Autodesk Fusion 360 part; units mm, degrees
note: some values were not read from the file. Chosen so that the rebuilt part matches the saved one: which face or edge a step refers to. Set by a fixed rule: which sketch regions a step uses.
(part 2 of 2)
sketch "Cap IV" plane through (0, 0, 30.6) normal (0, 0, 1) x (-1, 0, 0)
  circle A0 centre (-1.55, -2.515) radius 7.04 construction
  circle A1 centre (-1.55, -2.515) radius 7.405
  circle A2 centre (-1.55, -2.515) radius 7.24
  line L0 (5.6884, -2.365) -> (5.8535, -2.365) construction
  line L1 (5.69, -2.515) -> (5.855, -2.515) construction
  line L2 (5.6884, -2.665) -> (5.8535, -2.665) construction
  line L3 (-8.9535, -2.665) -> (-8.7884, -2.665) construction
  line L4 (-8.955, -2.515) -> (-8.79, -2.515) construction
  line L5 (-8.9535, -2.365) -> (-8.7884, -2.365) construction
  line L6 (-8.9535, -2.365) -> (-8.79, -2.515)
  line L7 (-8.9535, -2.665) -> (-8.79, -2.515)
  line L8 (5.8535, -2.365) -> (5.69, -2.515)
  line L9 (5.69, -2.515) -> (5.8535, -2.665)
  line L10 (-8.4473, -5.2096) -> (-8.2949, -5.1465) construction
  line L11 (-8.3913, -5.3488) -> (-8.2389, -5.2856) construction
  line L12 (5.1389, 0.2556) -> (5.2913, 0.3188) construction
  line L13 (-8.3325, -5.4868) -> (-8.18, -5.4236) construction
  line L14 (5.08, 0.3936) -> (5.2325, 0.4568) construction
  line L15 (5.1949, 0.1165) -> (5.3473, 0.1796) construction
  line L16 (5.2325, 0.4568) -> (5.1389, 0.2556)
  line L17 (5.1389, 0.2556) -> (5.3473, 0.1796)
  line L18 (-8.4473, -5.2096) -> (-8.2389, -5.2856)
  line L19 (-8.2389, -5.2856) -> (-8.3325, -5.4868)
  line L20 (3.4623, 2.7094) -> (3.579, 2.8261) construction
  line L21 (3.5695, 2.6045) -> (3.6861, 2.7211) construction
  line L22 (3.6744, 2.4973) -> (3.7911, 2.614) construction
  line L23 (-6.8911, -7.644) -> (-6.7744, -7.5273) construction
  line L24 (-6.7861, -7.7511) -> (-6.6695, -7.6345) construction
  line L25 (-6.679, -7.8561) -> (-6.5623, -7.7394) construction
  line L26 (-6.8911, -7.644) -> (-6.6695, -7.6345)
  line L27 (-6.6695, -7.6345) -> (-6.679, -7.8561)
  line L28 (3.579, 2.8261) -> (3.5695, 2.6045)
  line L29 (3.5695, 2.6045) -> (3.7911, 2.614)
  line L30 (1.0815, 4.2299) -> (1.1446, 4.3823) construction
  line L31 (1.2206, 4.1739) -> (1.2838, 4.3263) construction
  line L32 (1.3586, 4.115) -> (1.4218, 4.2675) construction
  line L33 (1.1446, 4.3823) -> (1.2206, 4.1739)
  line L34 (1.4218, 4.2675) -> (1.2206, 4.1739)
  line L35 (-4.5218, -9.2975) -> (-4.4586, -9.145) construction
  line L36 (-4.3838, -9.3563) -> (-4.3206, -9.2039) construction
  line L37 (-4.2446, -9.4123) -> (-4.1815, -9.2599) construction
  line L38 (-4.5218, -9.2975) -> (-4.3206, -9.2039)
  line L39 (-4.3206, -9.2039) -> (-4.2446, -9.4123)
  line L40 (-1.4, -9.9185) -> (-1.4, -9.7534) construction
  line L41 (-1.55, -9.92) -> (-1.55, -9.755) construction
  line L42 (-1.7, -9.9185) -> (-1.7, -9.7534) construction
  line L43 (-1.7, -9.9185) -> (-1.55, -9.755)
  line L44 (-1.55, -9.755) -> (-1.4, -9.9185)
  line L45 (-1.4, 4.7234) -> (-1.4, 4.8885) construction
  line L46 (-1.55, 4.725) -> (-1.55, 4.89) construction
  line L47 (-1.7, 4.7234) -> (-1.7, 4.8885) construction
  line L48 (-1.7, 4.8885) -> (-1.55, 4.725)
  line L49 (-1.55, 4.725) -> (-1.4, 4.8885)
  line L50 (1.1446, -9.4123) -> (1.0815, -9.2599) construction
  line L51 (1.2838, -9.3563) -> (1.2206, -9.2039) construction
  line L52 (1.4218, -9.2975) -> (1.3586, -9.145) construction
  line L53 (1.1446, -9.4123) -> (1.2206, -9.2039)
  line L54 (1.2206, -9.2039) -> (1.4218, -9.2975)
  line L55 (-4.4586, 4.115) -> (-4.5218, 4.2675) construction
  line L56 (-4.3206, 4.1739) -> (-4.3838, 4.3263) construction
  line L57 (-4.1815, 4.2299) -> (-4.2446, 4.3823) construction
  line L58 (-4.5218, 4.2675) -> (-4.3206, 4.1739)
  line L59 (-4.3206, 4.1739) -> (-4.2446, 4.3823)
  line L60 (3.579, -7.8561) -> (3.4623, -7.7394) construction
  line L61 (3.6861, -7.7511) -> (3.5695, -7.6345) construction
  line L62 (3.7911, -7.644) -> (3.6744, -7.5273) construction
  line L63 (3.579, -7.8561) -> (3.5695, -7.6345)
  line L64 (3.5695, -7.6345) -> (3.7911, -7.644)
  line L65 (-6.5623, 2.7094) -> (-6.679, 2.8261) construction
  line L66 (-6.6695, 2.6045) -> (-6.7861, 2.7211) construction
  line L67 (-6.7744, 2.4973) -> (-6.8911, 2.614) construction
  line L68 (-6.8911, 2.614) -> (-6.6695, 2.6045)
  line L69 (-6.6695, 2.6045) -> (-6.679, 2.8261)
  line L70 (5.2325, -5.4868) -> (5.08, -5.4236) construction
  line L71 (5.2913, -5.3488) -> (5.1389, -5.2856) construction
  line L72 (5.3473, -5.2096) -> (5.1949, -5.1465) construction
  line L73 (5.3473, -5.2096) -> (5.1389, -5.2856)
  line L74 (5.1389, -5.2856) -> (5.2325, -5.4868)
  line L75 (-8.2949, 0.1165) -> (-8.4473, 0.1796) construction
  line L76 (-8.2389, 0.2556) -> (-8.3913, 0.3188) construction
  line L77 (-8.18, 0.3936) -> (-8.3325, 0.4568) construction
  line L78 (-8.4473, 0.1796) -> (-8.2389, 0.2556)
  line L79 (-8.2389, 0.2556) -> (-8.3325, 0.4568)
  dimension "d129" = 0.2
  constraint horizontal L4
  constraint coincident A1 L2.end
  constraint coincident A1 L1.end
  constraint coincident A0.centre L4
  constraint collinear L0 L5
  constraint coincident A2 L0.start
  constraint coincident A2 L1.start
  constraint collinear L1 L4
  constraint collinear L2 L3
  constraint coincident A2 L2.start
  constraint coincident A1 L5.start
  constraint coincident A1 L4.start
  constraint coincident A1 L3.start
  constraint coincident A2 L3.end
  constraint coincident A2 L4.end
  constraint coincident A2 L5.end
  constraint coincident A1 L0.end
  constraint coincident A1 L15.end
  constraint coincident A1 L14.end
  constraint coincident A1 L12.end
  constraint coincident A1 L13.start
  constraint coincident A1 L11.start
  constraint coincident A1 L10.start
  constraint collinear L11 L12
  constraint coincident A2 L12.start
  constraint coincident A2 L14.start
  constraint coincident A2 L15.start
  constraint coincident A2 L10.end
  constraint coincident A2 L11.end
  constraint coincident A2 L13.end
  constraint coincident A2 L20.start
  constraint collinear L20 L23
  constraint coincident A2 L21.start
  constraint collinear L21 L24
  constraint coincident A2 L22.start
  constraint collinear L22 L25
  constraint coincident A1 L20.end
  constraint coincident A1 L21.end
  constraint coincident A1 L22.end
  constraint coincident A1 L23.start
  constraint coincident A1 L24.start
  constraint coincident A1 L25.start
  constraint coincident A2 L23.end
  constraint coincident A2 L24.end
  constraint coincident A2 L25.end
  constraint coincident A1 L32.end
  constraint coincident A1 L30.end
  constraint coincident A1 L31.end
  constraint coincident A2 L30.start
  constraint collinear L30 L35
  constraint coincident A2 L31.start
  constraint collinear L31 L36
  constraint coincident A2 L32.start
  constraint collinear L32 L37
  constraint coincident A1 L35.start
  constraint coincident A1 L36.start
  constraint coincident A1 L37.start
  constraint coincident A2 L35.end
  constraint coincident A2 L36.end
  constraint coincident A2 L37.end
  constraint coincident A1 L42.start
  constraint coincident A1 L40.start
  constraint coincident A1 L41.start
  constraint coincident A2 L40.end
  constraint coincident A2 L41.end
  constraint coincident A2 L42.end
  constraint coincident A1 L45.end
  constraint coincident A1 L47.end
  constraint coincident A1 L46.end
  constraint coincident A2 L45.start
  constraint coincident A2 L46.start
  constraint coincident A2 L47.start
  constraint coincident A1 L50.start
  constraint coincident A1 L52.start
  constraint coincident A1 L51.start
  constraint coincident A2 L50.end
  constraint coincident A2 L51.end
  constraint coincident A2 L52.end
  constraint coincident A1 L57.end
  constraint coincident A1 L55.end
  constraint coincident A1 L56.end
  constraint coincident A2 L55.start
  constraint coincident A2 L56.start
  constraint coincident A2 L57.start
  constraint coincident A1 L60.start
  constraint coincident A1 L62.start
  constraint coincident A1 L61.start
  constraint coincident A2 L60.end
  constraint coincident A2 L61.end
  constraint coincident A2 L62.end
  constraint coincident A1 L65.end
  constraint coincident A1 L67.end
  constraint coincident A1 L66.end
  constraint coincident A2 L65.start
  constraint coincident A2 L66.start
  constraint coincident A2 L67.start
  constraint coincident A1 L70.start
  constraint coincident A1 L72.start
  constraint coincident A1 L71.start
  constraint coincident A2 L70.end
  constraint coincident A2 L71.end
  constraint coincident A2 L72.end
  constraint coincident A1 L75.end
  constraint coincident A1 L77.end
  constraint coincident A1 L76.end
  constraint coincident A2 L75.start
  constraint coincident A2 L76.start
  constraint coincident A2 L77.start
extrude "Extrude22" cut sketch "Cap IV" against normal blind 14 contours A1 L8 L9 | A1 L16 L17 | A1 L73 L74 | A1 L28 L29 | A1 L63 L64 | A1 L33 L34 | A1 L53 L54 | A1 L48 L49 | A1 L43 L44 | A1 L58 L59 | A1 L38 L39 | A1 L68 L69 | A1 L26 L27 | A1 L78 L79 | A1 L18 L19 | A1 L6 L7 bodies 2
chamfer "Chamfer8" distance 0.25 angle 45 1 edges at (-5.0136, -0.0308, 30.6) on bodies 2
sketch "Cap V" plane through (0, 0, 30.6) normal (0, 0, 1) x (-1, 0, 0)
  circle A0 centre (-1.55, -2.515) radius 6.79
  line L0 (-1.55, -2.515) -> (-1.55, 4.275) construction
  line L1 (-1.55, 4.275) -> (-1.55, 2.275) construction
  line L2 (-1.8, 4.275) -> (-1.8, 2.275)
  line L3 (-1.35, 4.275) -> (-1.35, 2.275)
  line L4 (-1.35, 2.275) -> (-1.8, 2.275)
  line L5 (-1.35, 4.275) -> (-1.8, 4.275)
  line L6 (-1.8, 4.275) -> (-1.8, 4.7106)
  line L7 (-1.8, 4.7106) -> (-1.35, 4.7106)
  line L8 (-1.35, 4.7106) -> (-1.35, 4.275)
  dimension "d159" = 2
  dimension "d160" = 0.25
  dimension "d161" = -0.2
  constraint coincident A0.centre L0.start
  constraint coincident A0 L0.end
  constraint vertical L0
  constraint parallel L0 L1
  constraint perpendicular L2 L4
  constraint horizontal L5
  constraint vertical L6
  constraint horizontal L7
  constraint vertical L8
  measures "d159" distance of L0.end L1.end
extrude "Extrude23" cut sketch "Cap V" against normal blind 0.02 contours A0 L2 L3 L4 | L5 L6 L7 L8 picked at (-1.5667, 2.9417) bodies 2
extrude "Extrude24" cut 1 faces at (1.5, -2.275, 30.5933) along direction (0, -1, 0) blind 5.6 on bodies 2 bodies 2
sketch "Text" plane through (0, 0, 0) normal (0, 0, 1) x (-1, 0, 0)
  circle A0 centre (1.68, 4.535) radius 0.5 construction
  circle A1 centre (-4.78, 4.535) radius 0.5 construction
  circle A2 centre (-4.78, -10.115) radius 0.5 construction
  circle A3 centre (-1.55, -10.115) radius 0.5 construction
  circle A4 centre (1.68, -10.115) radius 0.5 construction
  circle A5 centre (-4.535, 10.35) radius 0.5 construction
  circle A6 centre (-2.025, 10.35) radius 0.5 construction
  circle A7 centre (-7.045, 10.35) radius 0.5 construction
  circle A8 centre (2.995, 10.35) radius 0.5 construction
  circle A9 centre (0.485, 10.35) radius 0.5 construction
  circle A10 centre (7, 8.075) radius 1.5 construction
  circle A11 centre (7, -8.775) radius 1.5 construction
  line L0 (-9.5, -13.125) -> (9.5, -13.125) construction
  line L1 (9.5, -13.125) -> (9.5, 13.125) construction
  line L2 (9.5, 13.125) -> (-9.5, 13.125) construction
  line L3 (-9.5, 13.125) -> (-9.5, -13.125) construction
  line L4 (9.5, 5.8343) -> (-9.5, 5.8343) construction
  line L5 (9.5, 8.775) -> (-9.5, 8.775) construction
  line L6 (-6.545, 8.775) -> (-6.545, 5.8343) construction
  line L7 (-4.035, 8.775) -> (-4.035, 5.8343) construction
  line L8 (-1.525, 8.775) -> (-1.525, 5.8343) construction
  line L9 (0.985, 8.775) -> (0.985, 5.8343) construction
  line L10 (3.495, 8.775) -> (3.495, 5.8343) construction
  dimension "d166" = -7.2907
  dimension "d167" = -4.35
  dimension "d168" = 0.85
  dimension "d169" = 0.85
  dimension "d170" = 0.85
  dimension "d171" = 1.25
  dimension "d172" = 0.85
  constraint coincident L4 L6.end
  constraint coincident L4 L7.end
  constraint coincident L4 L8.end
  constraint coincident L4 L9.end
  constraint coincident L4 L10.end
  constraint coincident L5 L6.start
  constraint coincident L5 L7.start
  constraint coincident L5 L8.start
  constraint coincident L5 L9.start
  constraint coincident L5 L10.start
equation "d9 = 4 mm - 2.45 mm"
equation "d11 = 1.2 mm + 12.55 mm"
equation "d118 = 14.080 mm - 0.55 mm - 0.55 mm"
equation "d124 = -16.60 mm + 4 mm"
named bodies: "Cap"

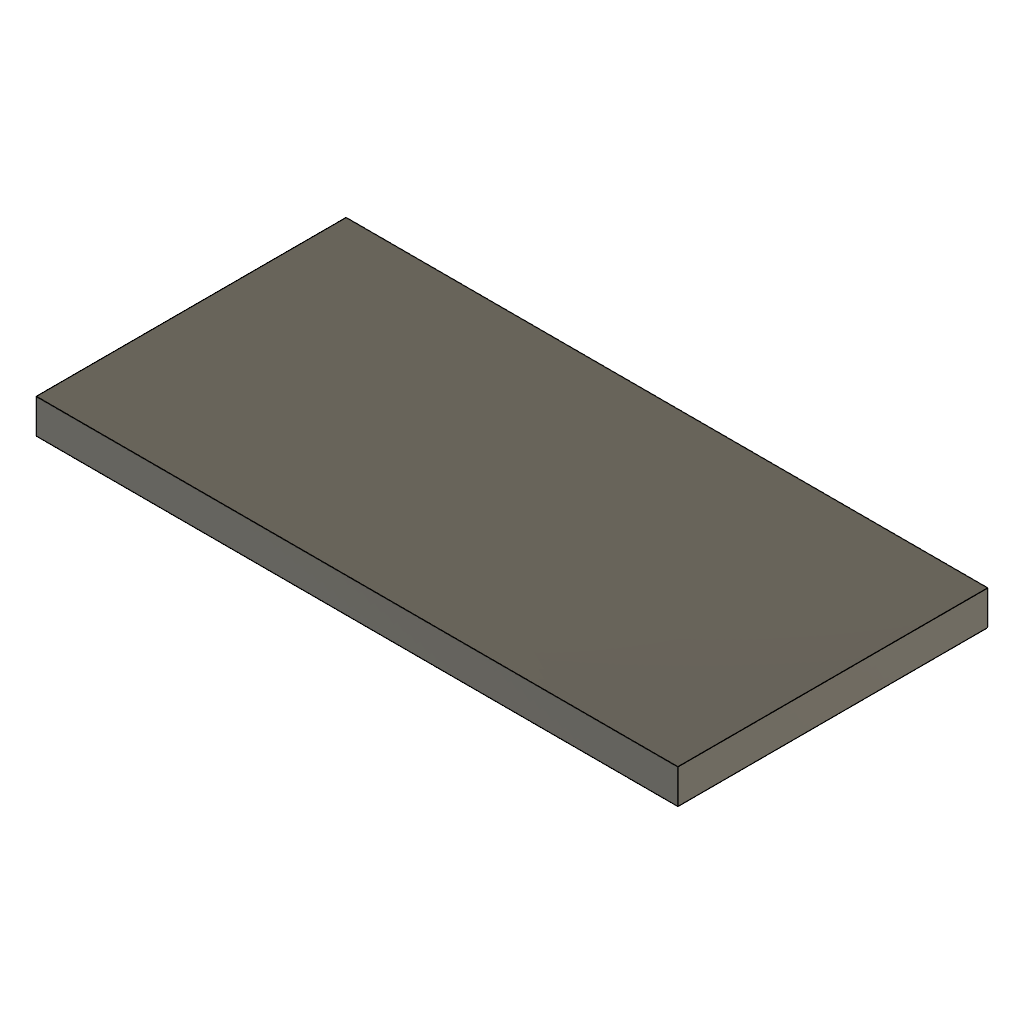
design "panel"
part number: 2026-09-25-18-54-46-307
Autodesk Fusion 360 part; units mm, degrees
sketch "Sketch1" plane through (0, 0, 0) normal (0, 0, 1) x (1, 0, 0)
  line L0 (13.975, 6.75) -> (-13.975, 6.75)
  line L1 (-13.975, 6.75) -> (-13.975, -6.75)
  line L2 (-13.975, -6.75) -> (13.975, -6.75)
  line L3 (13.975, -6.75) -> (13.975, 6.75)
  line L4 (13.975, 6.75) -> (-13.975, -6.75) construction
  line L5 (-13.975, 6.75) -> (13.975, -6.75) construction
  dimension "d1" = 27.95
  dimension "d2" = 13.5
  constraint horizontal L0
  constraint perpendicular L0 L1
  constraint parallel L0 L2
  constraint parallel L1 L3
  constraint coincident L4 origin
  constraint coincident L5 origin
  measures "d1" distance of L1.end L2.end
  measures "d2" distance of L0.end L1.end
extrude "Extrude1" add sketch "Sketch1" along normal blind 1.5

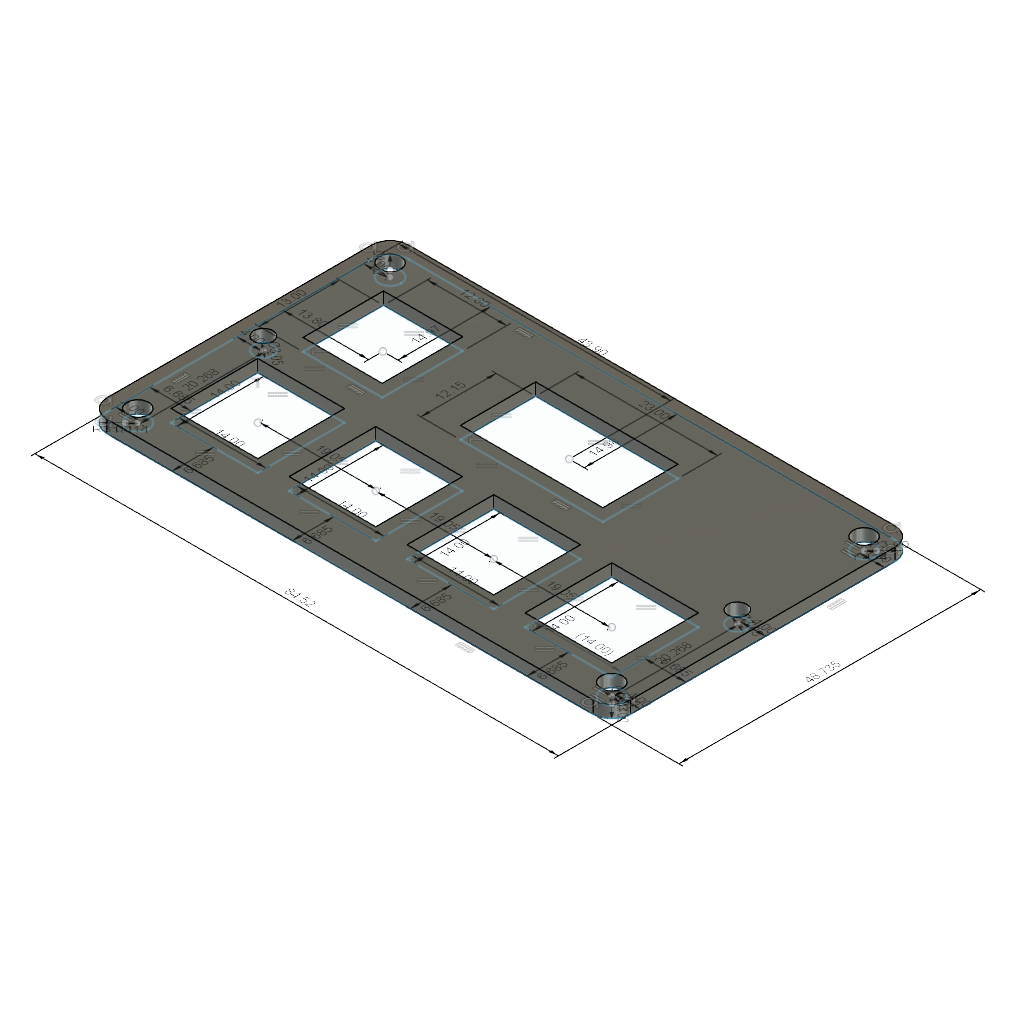
design "Hayai Top plate"
part number: 2026-09-20-15-53-54-702
Autodesk Fusion 360 part; units mm, degrees
sketch "Sketch1" plane through (0, 0, 0) normal (0, 0, 1) x (1, 0, 0)
  circle A0 centre (38.8472, 20.3675) radius 1.75
  circle A1 centre (38.8472, -0.0995) radius 1.525
  circle A2 centre (-37.6728, -20.3675) radius 1.75
  circle A3 centre (-37.6728, 20.3675) radius 1.75
  arc A4 (-38.6728, 24.3675) -> (-41.6728, 21.3675) centre (-38.6728, 21.3675) ccw
  line L0 (-38.6728, 24.3675) -> (39.8472, 24.3675)
  line L1 (-41.6728, -21.3675) -> (-41.6728, 21.3675)
  circle A5 centre (-37.6728, -0.0995) radius 1.525
  arc A6 (42.8472, 21.3675) -> (39.8472, 24.3675) centre (39.8472, 21.3675) ccw
  line L2 (42.8472, 21.3675) -> (42.8472, -21.3675)
  arc A7 (-41.6728, -21.3675) -> (-38.6728, -24.3675) centre (-38.6728, -21.3675) ccw
  line L3 (39.8472, -24.3675) -> (-38.6728, -24.3675)
  arc A8 (39.8472, -24.3675) -> (42.8472, -21.3675) centre (39.8472, -21.3675) ccw
  circle A9 centre (38.8472, -20.3675) radius 1.75
  line L4 (-20.9878, -3.6825) -> (-34.9878, -3.6825)
  line L5 (-34.9878, -3.6825) -> (-34.9878, -17.6825)
  line L6 (-34.9878, -17.6825) -> (-20.9878, -17.6825)
  line L7 (-20.9878, -17.6825) -> (-20.9878, -3.6825)
  line L8 (-1.9378, -17.6825) -> (-15.9378, -17.6825)
  line L9 (-15.9378, -17.6825) -> (-15.9378, -3.6825)
  line L10 (-15.9378, -3.6825) -> (-1.9378, -3.6825)
  line L11 (-1.9378, -3.6825) -> (-1.9378, -17.6825)
  line L12 (17.1122, -17.6825) -> (3.1122, -17.6825)
  line L13 (3.1122, -17.6825) -> (3.1122, -3.6825)
  line L14 (3.1122, -3.6825) -> (17.1122, -3.6825)
  line L15 (17.1122, -3.6825) -> (17.1122, -17.6825)
  line L16 (36.1622, -17.6825) -> (22.1622, -17.6825)
  line L17 (22.1622, -17.6825) -> (22.1622, -3.6825)
  line L18 (22.1622, -3.6825) -> (36.1622, -3.6825)
  line L19 (36.1622, -3.6825) -> (36.1622, -17.6825)
  line L20 (-21.4728, 2.8975) -> (-34.2728, 2.8975)
  line L21 (-34.2728, 2.8975) -> (-34.2728, 15.8975)
  line L22 (-34.2728, 15.8975) -> (-21.4728, 15.8975)
  line L23 (-21.4728, 15.8975) -> (-21.4728, 2.8975)
  line L24 (13.7272, 3.3125) -> (-9.2728, 3.3125)
  line L25 (-9.2728, 3.3125) -> (-9.2728, 15.4625)
  line L26 (-9.2728, 15.4625) -> (13.7272, 15.4625)
  line L27 (13.7272, 15.4625) -> (13.7272, 3.3125)
  point P0 (-27.9878, -10.6825)
  point P1 (-8.9378, -10.6825)
  point P2 (10.1122, -10.6825)
  point P3 (29.1622, -10.6825)
  point P4 (-27.8728, 9.3975)
  point P5 (2.2272, 9.3875)
  dimension "d44" = 3.05
  dimension "d45" = 3.05
  dimension "d46" = 20.268
  dimension "d47" = 3
  dimension "d48" = 3
  dimension "d49" = 3
  dimension "d50" = 3
  dimension "d51" = 3.5
  dimension "d52" = 4
  dimension "d53" = 1.4142
  dimension "d54" = 20.268
  dimension "d55" = 48.735
  dimension "d56" = 84.52
  dimension "d57" = 19.05
  dimension "d58" = 19.05
  dimension "d59" = 19.05
  dimension "d60" = 6.685
  dimension "d63" = 6.685
  dimension "d64" = 6.685
  dimension "d65" = 6.685
  dimension "d66" = 6.685
  dimension "d67" = 6.685
  dimension "d69" = 14
  dimension "d70" = 14
  dimension "d71" = 14
  dimension "d72" = 14
  dimension "d73" = 14
  dimension "d74" = 14
  dimension "d75" = 14
  dimension "d76" = 14
  dimension "d77" = 12.8
  dimension "d78" = 13
  dimension "d79" = 14.97
  dimension "d80" = 13.8
  dimension "d81" = 23
  dimension "d82" = 12.15
  dimension "d83" = 43.9
  dimension "d84" = 14.98
  dimension "d87" = 4
  dimension "d88" = 4
  dimension "d89" = 1.4142
  dimension "d92" = 4
  dimension "d93" = 1.4142
  dimension "d94" = 4
  dimension "d95" = 4
  constraint horizontal L0
  constraint vertical L2
  constraint horizontal L3
  constraint vertical L1
  constraint tangent A4 L0
  constraint tangent A4 L1
  constraint tangent L0 A6
  constraint tangent A6 L2
  constraint tangent L2 A8
  constraint tangent L3 A8
  constraint tangent A7 L3
  constraint tangent L1 A7
  constraint perpendicular L4 L5
  constraint parallel L4 L6
  constraint parallel L5 L7
  constraint perpendicular L8 L9
  constraint parallel L8 L10
  constraint parallel L9 L11
  constraint perpendicular L12 L13
  constraint parallel L12 L14
  constraint parallel L13 L15
  constraint perpendicular L16 L17
  constraint parallel L16 L18
  constraint parallel L17 L19
  constraint horizontal L20
  constraint perpendicular L20 L21
  constraint parallel L20 L22
  constraint parallel L21 L23
  constraint horizontal L24
  constraint perpendicular L24 L25
  constraint parallel L24 L26
  constraint parallel L25 L27
  constraint equal A0 A9
  constraint equal A0 A3
  constraint equal A2 A9
  measures "d44" diameter of A5
  measures "d45" diameter of A1
  measures "d46" distance of A5.centre A2.centre
  measures "d47" radius of A4
  measures "d48" radius of A6
  measures "d49" radius of A8
  measures "d50" radius of A7
  measures "d51" diameter of A9
  measures "d52" distance of L2 A9.centre
  measures "d53" distance of A8.centre A9.centre
  measures "d54" distance of A1.centre A9.centre
  measures "d55" distance of L0 L3
  measures "d56" distance of L1 L2
  measures "d57" distance of P0 P1
  measures "d58" distance of P1 P2
  measures "d59" distance of P2 P3
  measures "d60" distance of L2 L19
  measures "d63" distance of L1 L5
  measures "d64" distance of L3 L6
  measures "d65" distance of L3 L8
  measures "d66" distance of L3 L12
  measures "d67" distance of L3 L16
  measures "d69" distance of L4 L6
  measures "d70" distance of L5 L7
  measures "d71" distance of L9 L11
  measures "d72" distance of L8 L10
  measures "d73" distance of L12 L14
  measures "d74" distance of L13 L15
  measures "d75" distance of L16 L18
  measures "d76" distance of L17 L19
  measures "d77" distance of L21.end L22.end
  measures "d78" distance of L20.end L21.end
  measures "d79" distance of L0 P4
  measures "d80" distance of L1 P4
  measures "d81" distance of L25.end L26.end
  measures "d82" distance of L24.end L25.end
  measures "d83" distance of L1 P5
  measures "d84" distance of L0 P5
  measures "d87" distance of A3.centre L1
  measures "d88" distance of A0.centre L2
  measures "d89" distance of A0.centre A6.centre
  measures "d92" distance of A5.centre L1
  measures "d93" distance of A2.centre A7.centre
  measures "d94" distance of A2.centre L1
  measures "d95" distance of A1.centre L2
extrude "Extrude5" add sketch "Sketch1" along normal blind 2
extrude "Extrude1" [suppressed]
extrude "Extrude2" [suppressed]
extrude "Extrude3" [suppressed]
extrude "Extrude4" [suppressed]
equation "d53 = ( sqrt(2) ) * 1 mm"
equation "d89 = ( sqrt(2) ) * 1 mm"
